Autodesk Fusion 360 part; units mm, degrees
note: some values were not read from the file. Set by a fixed rule: which sketch regions a step uses.
(part 3 of 3)
sketch "plunger (2)" plane through (0, 0, 14.5) normal (0, 0, 1) x (-1, 0, 0) in component "plunger_5mm"
  circle A0 centre (-16, -54.7) radius 1.75
  circle A1 centre (-49.3, -12.8) radius 2.5 construction
  circle A2 centre (-20, -54.7) radius 1.75
  circle A3 centre (-24, -54.7) radius 1.75
  circle A4 centre (-28, -54.7) radius 1.75
  circle A5 centre (-12, -54.7) radius 1.75
  circle A6 centre (-8, -54.7) radius 1.75
  line L0 (-61.92, -3) -> (-61.92, -59.5)
  arc A7 (-61.92, -59.5) -> (-60.92, -60.5) centre (-60.92, -59.5) ccw
  line L1 (-60.92, -60.5) -> (8.8, -60.5)
  arc A8 (8.8, -60.5) -> (9.8, -59.5) centre (8.8, -59.5) ccw
  line L2 (9.8, -59.5) -> (9.8, -3)
  arc A9 (9.8, -3) -> (8.8, -2) centre (8.8, -3) ccw
  line L3 (8.8, -2) -> (-60.92, -2)
  arc A10 (-60.92, -2) -> (-61.92, -3) centre (-60.92, -3) ccw
  line L4 (-52.3, -10.5) -> (-52.3, -15.1) construction
  line L5 (-47, -9.8) -> (-51.6, -9.8)
  line L6 (-46.3, -15.1) -> (-46.3, -10.5) construction
  line L7 (-51.6, -15.8) -> (-47, -15.8)
  line L8 (-52.55, -11.35) -> (-52.05, -11.35) construction
  line L9 (-52.05, -14.25) -> (-52.55, -14.25) construction
  line L10 (-46.55, -14.25) -> (-46.05, -14.25) construction
  line L11 (-46.05, -11.35) -> (-46.55, -11.35) construction
  line L12 (-46.55, -11.35) -> (-46.55, -14.25) construction
  line L13 (-52.05, -11.35) -> (-52.05, -14.25) construction
  circle A11 centre (-49.3, -12.8) radius 2.5 construction
  line L14 (-52.3, -10.95) -> (-51.65, -10.95)
  line L15 (-51.65, -10.95) -> (-51.65, -14.65)
  line L16 (-51.65, -14.65) -> (-52.3, -14.65)
  line L17 (-46.3, -10.95) -> (-46.95, -10.95)
  line L18 (-46.95, -10.95) -> (-46.95, -14.65)
  line L19 (-46.95, -14.65) -> (-46.3, -14.65)
  line L20 (-52.3, -12.8) -> (-46.3, -12.8) construction
  line L21 (-49.3, -9.8) -> (-49.3, -15.8) construction
  line L22 (-52.3, -10.95) -> (-52.3, -10.5) construction
  line L23 (-52.3, -10.5) -> (-52.3, -10.95)
  line L24 (-52.3, -15.1) -> (-52.3, -14.65)
  line L25 (-46.3, -14.65) -> (-46.3, -15.1)
  line L26 (-46.3, -10.5) -> (-46.3, -10.95)
  circle A12 centre (-49.3, -12.8) radius 2.2
  line L27 (-46.3, -10.95) -> (-46.3, -14.65)
  line L28 (-52.3, -10.95) -> (-52.3, -14.65)
  arc A13 (-46.3, -10.5) -> (-47, -9.8) centre (-47, -10.5) ccw
  arc A14 (-51.6, -9.8) -> (-52.3, -10.5) centre (-51.6, -10.5) ccw
  arc A15 (-52.3, -15.1) -> (-51.6, -15.8) centre (-51.6, -15.1) ccw
  arc A16 (-47, -15.8) -> (-46.3, -15.1) centre (-47, -15.1) ccw
  dimension "d132_1" = 0.4
  dimension "d133_1" = 0.4
  dimension "d134_1" = 4.4
  dimension "d139_1" = 0.7
  dimension "d142_1" = 0.4
  constraint coincident L4 L14.start
  constraint perpendicular L4 L14
  constraint perpendicular L14 L15
  constraint coincident L4 L16.end
  constraint perpendicular L4 L16
  constraint coincident L6 L17.start
  constraint perpendicular L6 L17
  constraint perpendicular L17 L18
  constraint coincident L6 L19.end
  constraint perpendicular L6 L19
  constraint symmetric L15 L18 L21
  constraint symmetric L16 L19 L21
  constraint symmetric L14 L17 L21
  constraint concentric A11 A12
  constraint coincident L6 L20.end
  constraint coincident L5 L21.start
  constraint tangent L6 A13
  constraint tangent L5 A13
  constraint coincident L4 L20.start
  constraint tangent L5 A14
  constraint tangent L4 A14
  constraint equal A13 A14
  constraint coincident L7 L21.end
  constraint tangent L7 A15
  constraint tangent L4 A15
  constraint equal A13 A15
  constraint tangent L7 A16
  constraint tangent L6 A16
  constraint equal A13 A16
  constraint symmetric L21 L23 L26
  measures "d132_1" distance of L8 L14
  measures "d133_1" distance of L13 L15
  measures "d134_1" diameter of A12
  measures "d139_1" radius of A13
  measures "d142_1" distance of L9 L16
extrude "Extrude1''''" add sketch "plunger (2)" along normal blind 3 and the other way blind 0.5 separate body contours A12 makes body 14 in component "plunger_5mm"
extrude "Extrude2''''" add sketch "plunger (2)" against normal blind 4 from surface at -0.5 separate body contours L17 L18 L19 L27 | L14 L15 L16 L28 makes body 15 at (46.3, 12.1833, 12.6667) makes body 16 at (52.3, 12.1833, 12.6667) in component "plunger_5mm"
extrude "Extrude3''''" add sketch "plunger (2)" against normal blind 6.5 from surface at -0.5 contours L5 L7 L14 L15 L16 L17 L18 L19 L23 L24 L25 L26 A13 A14 A15 A16 | A12 bodies 14 15 16 in component "plunger_5mm"
move_face "OffsetFaces1" offset 2 1 faces at (50.0833, 12.1833, 7.5) on bodies 14 in component "plunger_5mm"
sketch "plunger (3)" plane through (0, 0, 14.5) normal (0, 0, 1) x (-1, 0, 0) in component "plunger_4mm"
  circle A0 centre (-16, -54.7) radius 1.75
  circle A1 centre (-49.3, -12.8) radius 2.5 construction
  circle A2 centre (-20, -54.7) radius 1.75
  circle A3 centre (-24, -54.7) radius 1.75
  circle A4 centre (-28, -54.7) radius 1.75
  circle A5 centre (-12, -54.7) radius 1.75
  circle A6 centre (-8, -54.7) radius 1.75
  line L0 (-61.92, -3) -> (-61.92, -59.5)
  arc A7 (-61.92, -59.5) -> (-60.92, -60.5) centre (-60.92, -59.5) ccw
  line L1 (-60.92, -60.5) -> (8.8, -60.5)
  arc A8 (8.8, -60.5) -> (9.8, -59.5) centre (8.8, -59.5) ccw
  line L2 (9.8, -59.5) -> (9.8, -3)
  arc A9 (9.8, -3) -> (8.8, -2) centre (8.8, -3) ccw
  line L3 (8.8, -2) -> (-60.92, -2)
  arc A10 (-60.92, -2) -> (-61.92, -3) centre (-60.92, -3) ccw
  line L4 (-52.3, -10.5) -> (-52.3, -15.1) construction
  line L5 (-47, -9.8) -> (-51.6, -9.8)
  line L6 (-46.3, -15.1) -> (-46.3, -10.5) construction
  line L7 (-51.6, -15.8) -> (-47, -15.8)
  line L8 (-52.55, -11.35) -> (-52.05, -11.35) construction
  line L9 (-52.05, -14.25) -> (-52.55, -14.25) construction
  line L10 (-46.55, -14.25) -> (-46.05, -14.25) construction
  line L11 (-46.05, -11.35) -> (-46.55, -11.35) construction
  line L12 (-46.55, -11.35) -> (-46.55, -14.25) construction
  line L13 (-52.05, -11.35) -> (-52.05, -14.25) construction
  circle A11 centre (-49.3, -12.8) radius 2.5 construction
  line L14 (-52.3, -10.95) -> (-51.65, -10.95)
  line L15 (-51.65, -10.95) -> (-51.65, -14.65)
  line L16 (-51.65, -14.65) -> (-52.3, -14.65)
  line L17 (-46.3, -10.95) -> (-46.95, -10.95)
  line L18 (-46.95, -10.95) -> (-46.95, -14.65)
  line L19 (-46.95, -14.65) -> (-46.3, -14.65)
  line L20 (-52.3, -12.8) -> (-46.3, -12.8) construction
  line L21 (-49.3, -9.8) -> (-49.3, -15.8) construction
  line L22 (-52.3, -10.95) -> (-52.3, -10.5) construction
  line L23 (-52.3, -10.5) -> (-52.3, -10.95)
  line L24 (-52.3, -15.1) -> (-52.3, -14.65)
  line L25 (-46.3, -14.65) -> (-46.3, -15.1)
  line L26 (-46.3, -10.5) -> (-46.3, -10.95)
  circle A12 centre (-49.3, -12.8) radius 2.2
  line L27 (-46.3, -10.95) -> (-46.3, -14.65)
  line L28 (-52.3, -10.95) -> (-52.3, -14.65)
  arc A13 (-46.3, -10.5) -> (-47, -9.8) centre (-47, -10.5) ccw
  arc A14 (-51.6, -9.8) -> (-52.3, -10.5) centre (-51.6, -10.5) ccw
  arc A15 (-52.3, -15.1) -> (-51.6, -15.8) centre (-51.6, -15.1) ccw
  arc A16 (-47, -15.8) -> (-46.3, -15.1) centre (-47, -15.1) ccw
  dimension "d132_2" = 0.4
  dimension "d133_2" = 0.4
  dimension "d134_2" = 4.4
  dimension "d139_2" = 0.7
  dimension "d142_2" = 0.4
  constraint coincident L4 L14.start
  constraint perpendicular L4 L14
  constraint perpendicular L14 L15
  constraint coincident L4 L16.end
  constraint perpendicular L4 L16
  constraint coincident L6 L17.start
  constraint perpendicular L6 L17
  constraint perpendicular L17 L18
  constraint coincident L6 L19.end
  constraint perpendicular L6 L19
  constraint symmetric L15 L18 L21
  constraint symmetric L16 L19 L21
  constraint symmetric L14 L17 L21
  constraint concentric A11 A12
  constraint coincident L6 L20.end
  constraint coincident L5 L21.start
  constraint tangent L6 A13
  constraint tangent L5 A13
  constraint coincident L4 L20.start
  constraint tangent L5 A14
  constraint tangent L4 A14
  constraint equal A13 A14
  constraint coincident L7 L21.end
  constraint tangent L7 A15
  constraint tangent L4 A15
  constraint equal A13 A15
  constraint tangent L7 A16
  constraint tangent L6 A16
  constraint equal A13 A16
  constraint symmetric L21 L23 L26
  measures "d132_2" distance of L8 L14
  measures "d133_2" distance of L13 L15
  measures "d134_2" diameter of A12
  measures "d139_2" radius of A13
  measures "d142_2" distance of L9 L16
extrude "Extrude1'''''" add sketch "plunger (3)" along normal blind 3 and the other way blind 0.5 separate body contours A12 makes body 17 in component "plunger_4mm"
extrude "Extrude2'''''" add sketch "plunger (3)" against normal blind 4 from surface at -0.5 separate body contours L17 L18 L19 L27 | L14 L15 L16 L28 makes body 18 at (46.3, 12.1833, 12.6667) makes body 19 at (52.3, 12.1833, 12.6667) in component "plunger_4mm"
extrude "Extrude3'''''" add sketch "plunger (3)" against normal blind 6.5 from surface at -0.5 contours L5 L7 L14 L15 L16 L17 L18 L19 L23 L24 L25 L26 A13 A14 A15 A16 | A12 bodies 17 18 19 in component "plunger_4mm"
move_face "OffsetFaces1'" offset 3 1 faces at (50.0833, 12.1833, 7.5) on bodies 17 in component "plunger_4mm"
component "PCB" placed x (1, 0, 0) y (0, 1, 0) z (0, 0, 1) at (0, 0, 0)
component "C64_WiFi2_Top" placed x (1, 0, 0) y (0, 1, 0) z (0, 0, 1) at (0, 0, 0)
component "C64_Wifi2_bottom" placed x (1, 0, 0) y (0, 1, 0) z (0, 0, 1) at (0, 0, 0)
component "plunger_7mm" placed x (1, 0, 0) y (0, 1, 0) z (0, 0, 1) at (0, 0, 0)
component "plunger_5mm" placed x (1, 0, 0) y (0, 1, 0) z (0, 0, 1) at (39, 0, 0)
component "plunger_4mm" placed x (1, 0, 0) y (0, 1, 0) z (0, 0, 1) at (39, 10, 0)
equation "wall = 2 mm"
equation "above = 16.5 mm"
equation "below = 6.6 mm"
equation "tolerance = 0.3 mm"
equation "d28 = above - wall"
equation "d29 = -below + wall"
equation "corner_rnd = 3 mm"
equation "wall_dist = 1.5 mm"
equation "d32 = corner_rnd"
equation "d33 = corner_rnd"
equation "d34 = wall_dist + wall"
equation "d35 = wall_dist + wall"
equation "d36 = wall"
equation "d38 = tolerance"
equation "d39 = tolerance"
equation "d40 = 0.6 * wall"
equation "d53 = tolerance"
equation "d54 = d52"
equation "d55 = d50"
equation "d56 = d51"
equation "d57 = d55 / 2"
equation "d58 = tolerance"
equation "seam_level = 4.5 mm"
equation "d60 = -wall"
equation "d62 = below - wall - 1.6 mm"
equation "d64 = below - wall"
equation "d67 = below - wall - 1.6 mm - 1 mm"
equation "overlap = 1 mm"
equation "d70 = below - wall + seam_level + overlap"
equation "d72 = below - wall + seam_level"
equation "d77 = wall * 0.4"
equation "d78 = led"
equation "d79 = led"
equation "led = 3.5 mm"
equation "d81 = led"
equation "d82 = led"
equation "d83 = led"
equation "d84 = led"
equation "d86 = d85"
equation "plungersquare = 6 mm"
equation "d89 = plungersquare"
equation "d90 = plungersquare"
equation "d95 = plungersquare + 0.7 mm"
equation "d96 = plungersquare + 0.7 mm"
equation "d97 = plungersquare + 2.7 mm"
equation "d98 = plungersquare + 2.7 mm"
equation "d100 = d99"
equation "d101 = d99"
equation "d102 = d99"
equation "d103 = d99"
equation "d104 = d99"
equation "d105 = d99"
equation "d106 = d99"
equation "d108 = d107"
equation "d111 = wall"
equation "d113 = -above + wall + overlap + tolerance + seam_level"
equation "d115 = -above + wall + tolerance + seam_level"
equation "d119 = -above + wall"
equation "pl_frame_height = 7 mm"
equation "d122 = -pl_frame_height"
equation "d125 = -pl_frame_height + 1.5 mm"
equation "d133 = tolerance + 0.1 mm"
equation "d135 = wall + 1 mm"
equation "d137 = -pl_frame_height + 3 mm"
equation "d140 = -above + wall + 8 mm"
equation "d133_1 = tolerance + 0.1 mm"
equation "d135_1 = wall + 1 mm"
equation "d137_1 = -pl_frame_height + 3 mm"
equation "d140_1 = -above + wall + 8 mm"
equation "d133_2 = tolerance + 0.1 mm"
equation "d135_2 = wall + 1 mm"
equation "d137_2 = -pl_frame_height + 3 mm"
equation "d140_2 = -above + wall + 8 mm"
named bodies: "pcb", "bottom shell", "top shell", "plunger"
